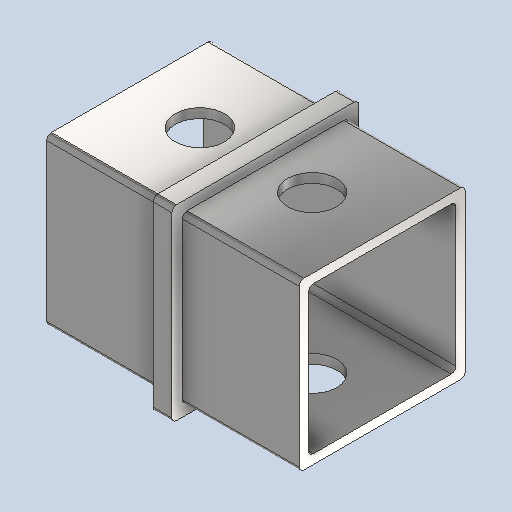
# Autodesk Inventor part: Verbinder
Saved by Autodesk Inventor 2024.4 (Build 284460000, 460)
## iProperties
Created: 2026-01-10
Part Number: Verbinder
Material: Edelstahl, 440C
Description: Verbinder
Document SubType Name: Modeling
Designer: Al Hefawi
Mass: 117.322 g
Surface Area: 151.453 cm^2
Volume: 15.1383 cm^3
Density: 7.75 g/cm^3
Appearance: Halbpoliert
DocNumber: Verbinder.ipt
Folder: I60-Konstruktion\I60-Gruppe-7\Gestell\
VDS_Category: Konstruktion
Masse[kg]: 0,015 kg
Comments: wird gekauft
Autodesk Inventor part; units mm, degrees
ref_plane "YZ Plane" through (0, 0, 0) normal (1, 0, 0) x (0, 1, 0)
ref_plane "XZ Plane" through (0, 0, 0) normal (0, 1, 0) x (-1, 0, 0)
ref_plane "XY Plane" through (0, 0, 0) normal (0, 0, 1) x (1, 0, 0)
sketch "Skizze1" plane through (0, 0, 0) normal (1, 0, 0) x (0, 1, 0)
  line L0 (-16.75, 17.75) -> (16.75, 17.75)
  line L1 (17.75, 16.75) -> (17.75, -16.75)
  line L2 (16.75, -17.75) -> (-16.75, -17.75)
  line L3 (-17.75, -16.75) -> (-17.75, 16.75)
  line L4 (-17.75, 17.75) -> (17.75, -17.75) construction
  line L5 (17.75, 17.75) -> (-17.75, -17.75) construction
  line L6 (-14.75, 15.75) -> (14.75, 15.75)
  line L7 (15.75, 14.75) -> (15.75, -14.75)
  line L8 (14.75, -15.75) -> (-14.75, -15.75)
  line L9 (-15.75, -14.75) -> (-15.75, 14.75)
  line L10 (-15.75, 15.75) -> (15.75, -15.75) construction
  line L11 (15.75, 15.75) -> (-15.75, -15.75) construction
  arc A0 (17.75, 16.75) -> (16.75, 17.75) centre (16.75, 16.75) ccw
  arc A1 (-16.75, 17.75) -> (-17.75, 16.75) centre (-16.75, 16.75) ccw
  arc A2 (-17.75, -16.75) -> (-16.75, -17.75) centre (-16.75, -16.75) ccw
  arc A3 (16.75, -17.75) -> (17.75, -16.75) centre (16.75, -16.75) ccw
  arc A4 (14.75, -15.75) -> (15.75, -14.75) centre (14.75, -14.75) ccw
  arc A5 (-15.75, -14.75) -> (-14.75, -15.75) centre (-14.75, -14.75) ccw
  arc A6 (-14.75, 15.75) -> (-15.75, 14.75) centre (-14.75, 14.75) ccw
  arc A7 (15.75, 14.75) -> (14.75, 15.75) centre (14.75, 14.75) ccw
  point P0 (0, 0)
  dimension "d0" = 35.5
  dimension "d1" = 35.5
  dimension "d2" = 31.5
  dimension "d3" = 31.5
  dimension "d4" = 1
  constraints: 24 end point, 16 point on circle, 16 point on line, 16 tangent, 8 centre point, 7 equal radius, 4 midpoint, 4 parallel, 2 horizontal, 2 perpendicular
  measures "d0" distance of L4.end L5.end
  measures "d1" distance of L5.start L4.end
  measures "d2" distance of L10.end L11.end
  measures "d3" distance of L11.start L10.end
  measures "d4" radius of A0
extrude "Extrusion1" add sketch "Skizze1" along normal blind 25
sketch "Skizze2" plane through (0, 0, 0) normal (-1, 0, 0) x (0, 0, 1)
  line L0 (19, 20) -> (-19, 20)
  line L1 (-20, 19) -> (-20, -19)
  line L2 (-19, -20) -> (19, -20)
  line L3 (20, -19) -> (20, 19)
  line L4 (20, 20) -> (-20, -20) construction
  line L5 (-20, 20) -> (20, -20) construction
  line L6 (16.75, 17.75) -> (-16.75, 17.75)
  line L7 (-17.75, 16.75) -> (-17.75, -16.75)
  line L8 (-16.75, -17.75) -> (16.75, -17.75)
  line L9 (17.75, -16.75) -> (17.75, 16.75)
  line L10 (17.75, 17.75) -> (-17.75, -17.75) construction
  line L11 (-17.75, 17.75) -> (17.75, -17.75) construction
  arc A0 (19, -20) -> (20, -19) centre (19, -19) ccw
  arc A1 (20, 19) -> (19, 20) centre (19, 19) ccw
  arc A2 (-19, 20) -> (-20, 19) centre (-19, 19) ccw
  arc A3 (-20, -19) -> (-19, -20) centre (-19, -19) ccw
  arc A4 (-17.75, -16.75) -> (-16.75, -17.75) centre (-16.75, -16.75) ccw
  arc A5 (-16.75, 17.75) -> (-17.75, 16.75) centre (-16.75, 16.75) ccw
  arc A6 (17.75, 16.75) -> (16.75, 17.75) centre (16.75, 16.75) ccw
  arc A7 (16.75, -17.75) -> (17.75, -16.75) centre (16.75, -16.75) ccw
  line L12 (-16.75, 17.75) -> (16.75, 17.75)
  line L13 (17.75, 16.75) -> (17.75, -16.75)
  line L14 (16.75, -17.75) -> (-16.75, -17.75)
  line L15 (-17.75, -16.75) -> (-17.75, 16.75)
  line L16 (-17.75, 17.75) -> (17.75, -17.75) construction
  line L17 (17.75, 17.75) -> (-17.75, -17.75) construction
  arc A8 (17.75, 16.75) -> (16.75, 17.75) centre (16.75, 16.75) ccw
  arc A9 (17.75, 16.75) -> (16.75, 17.75) centre (16.75, 16.75) ccw
  arc A10 (16.75, -17.75) -> (17.75, -16.75) centre (16.75, -16.75) ccw
  arc A11 (-16.75, 17.75) -> (-17.75, 16.75) centre (-16.75, 16.75) ccw
  arc A12 (-17.75, -16.75) -> (-16.75, -17.75) centre (-16.75, -16.75) ccw
  point P0 (0, 0)
  dimension "d7" = 40
  dimension "d8" = 40
  dimension "d9" = 1
  dimension "d10" = 1
  dimension "d11" = 1
  constraints: 36 end point, 27 point on line, 26 point on circle, 26 tangent, 13 centre point, 10 equal radius, 6 midpoint, 6 parallel, 3 horizontal, 3 perpendicular
  measures "d7" distance of L5.end L4.end
  measures "d8" distance of L4.end L5.start
  measures "d9" radius of A0
  measures "d10" radius of A4
  measures "d11" radius of A8
extrude "Extrusion2" add sketch "Skizze2" along normal blind 4 contours A1 L3 A0 L2 A3 L1 A2 L0 | A6 L9 A7 L8 A4 L7 A5 L6
sketch "Skizze3" plane through (-4, 0, 0) normal (-1, 0, 0) x (0, 0, 1)
  line L0 (-14.75, 15.75) -> (14.75, 15.75)
  line L1 (15.75, 14.75) -> (15.75, -14.75)
  line L2 (14.75, -15.75) -> (-14.75, -15.75)
  line L3 (-15.75, -14.75) -> (-15.75, 14.75)
  line L4 (-15.75, 15.75) -> (15.75, -15.75) construction
  line L5 (15.75, 15.75) -> (-15.75, -15.75) construction
  arc A0 (15.75, 14.75) -> (14.75, 15.75) centre (14.75, 14.75) ccw
  arc A1 (-14.75, 15.75) -> (-15.75, 14.75) centre (-14.75, 14.75) ccw
  arc A2 (-15.75, -14.75) -> (-14.75, -15.75) centre (-14.75, -14.75) ccw
  arc A3 (14.75, -15.75) -> (15.75, -14.75) centre (14.75, -14.75) ccw
  point P0 (0, 0)
  dimension "d14" = 31.5
  dimension "d15" = 1
  constraints: 12 end point, 8 point on circle, 8 point on line, 8 tangent, 4 centre point, 3 equal radius, 2 midpoint, 2 parallel, 1 horizontal, 1 perpendicular
  measures "d14" distance of L4.end L5.end
  measures "d15" radius of A0
extrude "Extrusion3" cut sketch "Skizze3" against normal blind 4
sketch "Skizze4" plane through (-4, 0, 0) normal (-1, 0, 0) x (0, 0, 1)
  line L0 (-16.75, 17.75) -> (16.75, 17.75)
  line L1 (17.75, 16.75) -> (17.75, -16.75)
  line L2 (16.75, -17.75) -> (-16.75, -17.75)
  line L3 (-17.75, -16.75) -> (-17.75, 16.75)
  line L4 (-17.75, 17.75) -> (17.75, -17.75) construction
  line L5 (17.75, 17.75) -> (-17.75, -17.75) construction
  line L6 (-14.75, 15.75) -> (14.75, 15.75)
  line L7 (15.75, 14.75) -> (15.75, -14.75)
  line L8 (14.75, -15.75) -> (-14.75, -15.75)
  line L9 (-15.75, -14.75) -> (-15.75, 14.75)
  line L10 (-15.75, 15.75) -> (15.75, -15.75) construction
  line L11 (15.75, 15.75) -> (-15.75, -15.75) construction
  arc A0 (17.75, 16.75) -> (16.75, 17.75) centre (16.75, 16.75) ccw
  arc A1 (16.75, -17.75) -> (17.75, -16.75) centre (16.75, -16.75) ccw
  arc A2 (-17.75, -16.75) -> (-16.75, -17.75) centre (-16.75, -16.75) ccw
  arc A3 (-16.75, 17.75) -> (-17.75, 16.75) centre (-16.75, 16.75) ccw
  arc A4 (-14.75, 15.75) -> (-15.75, 14.75) centre (-14.75, 14.75) ccw
  arc A5 (15.75, 14.75) -> (14.75, 15.75) centre (14.75, 14.75) ccw
  arc A6 (14.75, -15.75) -> (15.75, -14.75) centre (14.75, -14.75) ccw
  arc A7 (-15.75, -14.75) -> (-14.75, -15.75) centre (-14.75, -14.75) ccw
  point P0 (0, 0)
  dimension "d18" = 1
  constraints: 24 end point, 17 point on line, 16 point on circle, 16 tangent, 8 centre point, 7 equal radius, 4 midpoint, 4 parallel, 2 horizontal, 2 perpendicular
  measures "d18" radius of A0
extrude "Extrusion4" add sketch "Skizze4" along normal blind 25
sketch "Skizze5" plane through (25, -16.75, 17.75) normal (0, 0, 1) x (1, 0, 0)
  line L0 (-25, 16.75) -> (-15, 16.75)
  line L1 (-15, 16.75) -> (-39, 16.75)
  circle A0 centre (-15, 16.75) radius 5.25
  circle A1 centre (-39, 16.75) radius 5.25
  dimension "d21" = 10
  dimension "d22" = 24
  dimension "d23" = 10.5
  dimension "d24" = 10.5
  constraints: 4 end point, 2 centre point, 2 coincident, 1 horizontal, 1 point on line
  measures "d21" distance of L0.start L0.end
  measures "d22" distance of L0.end L1.end
  measures "d23" diameter of A0
  measures "d24" diameter of A1
extrude "Extrusion5" cut sketch "Skizze5" against normal blind 50
